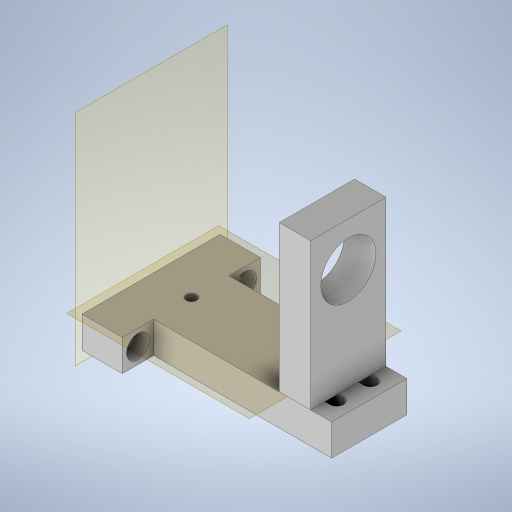
# Autodesk Inventor part: AdapterBracket
Saved by Autodesk Inventor 2024 (Build 280153000, 153)
## iProperties
Created: 2026-02-24
Part Number: AdapterBracket
Material: Generic
Document SubType Name: Modeling
Designer: nvladi
Density: 1 g/cm^3
Appearance: Default
Author: nvladi
Autodesk Inventor part; units mm, degrees
ref_plane "YZ Plane" through (0, 0, 0) normal (1, 0, 0) x (0, 1, 0)
ref_plane "XZ Plane" through (0, 0, 0) normal (0, 1, 0) x (-1, 0, 0)
ref_plane "Work Plane1" through (0, 0, 0) normal (0, 0, 1) x (1, 0, 0)
sketch "Sketch1" plane through (0, 0, 0) normal (0, 0, 1) x (1, 0, 0)
  line L0 (2, 95.25) -> (68, 95.25)
  line L1 (2, 80.25) -> (68, 80.25)
  line L2 (2, 0) -> (2, 95.25)
  line L3 (68, 95.25) -> (68, 0)
  point P0 (0, 0)
  constraints: 8 end point, 2 horizontal, 2 vertical, 6 other
ref_plane "Work Plane2" through (12.0686, 8.3392, 79.2624) normal (0, 0, 1) x (1, 0, 0)
extrude "Extrusion1" add sketch "Sketch1" along normal up to surface (79.2624 mm away)
sketch "Sketch2" plane through (2, 95.25, 79.2624) normal (0, 0, 1) x (1, 0, 0)
  line L0 (66, -15) -> (66, 0) projected
  line L1 (66, 0) -> (0, 0) projected
  line L2 (66, -15) -> (51, -15)
  line L3 (51, -15) -> (51, 0)
  line L4 (51, 0) -> (66, 0)
  line L5 (66, 0) -> (66, -15)
  line L6 (0, 0) -> (0, -15) projected
  line L7 (0, -15) -> (15, -15)
  line L8 (15, -15) -> (15, 0)
  line L9 (15, 0) -> (0, 0)
  line L10 (0, 0) -> (0, -15)
  point P0 (-2, -95.25)
  dimension "d2" = 15
  dimension "d3" = 15
  constraints: 16 end point, 4 parallel, 2 horizontal, 2 perpendicular, 2 point on line
  measures "d2" distance of L3.end L4.end
  measures "d3" distance of L9.end L8.end
extrude "Extrusion2" cut sketch "Sketch2" against normal blind 60
sketch "Sketch4" plane through (2, 95.25, 19.2624) normal (0, 0, 1) x (1, 0, 0)
  line L0 (66, -15) -> (51, -15) projected
  line L1 (66, 0) -> (66, -15) projected
  line L2 (51, 0) -> (66, 0) projected
  line L3 (51, -15) -> (51, 0) projected
  line L4 (15, -15) -> (0, -15) projected
  line L5 (0, -15) -> (0, 0) projected
  line L6 (15, 0) -> (15, -15) projected
  line L7 (0, 0) -> (15, 0) projected
  point P0 (-2, -95.25)
  point P1 (58.5, -7.5)
  point P2 (7.5, -7.5)
hole "Hole1" at (60.5, 87.75, 19.2624) at (9.5, 87.75, 19.2624) direction (0, 0, -1) diameter 6.6 end through all counterbore diameter 11 counterbore depth 6.8 clearance for "Socket Head Cap Screw ISO 4762" size "M6" standard "ISO"
sketch "Sketch5" plane through (2, 95.25, 0) normal (0, 1, 0) x (1, 0, 0)
  line L0 (51, -79.2624) -> (51, -19.2624) projected
  line L1 (15, -19.2624) -> (15, -79.2624) projected
  line L2 (15, -79.2624) -> (51, -79.2624) projected
  line L3 (51, -79.2624) -> (15, -79.2624)
  line L4 (15, -79.2624) -> (15, -94.2624)
  line L5 (15, -94.2624) -> (51, -94.2624)
  line L6 (51, -94.2624) -> (51, -79.2624)
  point P0 (-2, 0)
  dimension "d13" = 15
  constraints: 8 end point, 2 parallel, 1 horizontal, 1 perpendicular
  measures "d13" distance of L4.end L3.end
extrude "Extrusion3" add sketch "Sketch5" against normal blind 85
sketch "Sketch6" plane through (17, 95.25, 94.2624) normal (0, 0, 1) x (1, 0, 0)
  circle A0 centre (18, -64) radius 25
  circle A1 centre (18, -64) radius 13.1445
  point P0 (-17, -95.25)
  dimension "d16" = 26.289
  constraints: 2 centre point, 1 coincident, 2 other
  measures "d16" diameter of A1
extrude "Extrusion4" cut sketch "Sketch6" against normal up to surface (15 mm away) contours A1
sketch "Sketch7" plane through (2, 95.25, 0) normal (0, 1, 0) x (1, 0, 0)
  line L0 (66, 0) -> (0, 0) projected
  line L1 (51, -94.2624) -> (51, -19.2624) projected
  line L2 (15, -19.2624) -> (15, -94.2624) projected
  line L3 (15, -94.2624) -> (51, -94.2624) projected
  line L4 (51, -94.2624) -> (51, -19.2624) projected
  line L5 (51, -19.2624) -> (66, -19.2624) projected
  line L6 (66, 0) -> (66, -19.2624) projected
  line L7 (66, 0) -> (0, 0) projected
  line L8 (0, 0) -> (0, -19.2624) projected
  line L9 (0, -19.2624) -> (15, -19.2624) projected
  point P0 (-2, 0)
  point P1 (33, -19.2624)
  point P2 (33, -69.2624)
  dimension "d19" = 50
  constraints: 1 other
  measures "d19" distance of point (33, -69.262) point (33, -19.262)
hole "Hole2" at (35, 95.25, 19.2624) at (35, 95.25, 69.2624) direction (0, -1, 0) diameter 4.9784 depth 19.05 tip angle 118 thread size "1/4-20 UNC" class "2B" standard "ANSI Unified Screw Threads"
ref_plane "Work Plane3" through (2, 80.25, 0) normal (0, -1, 0) x (1, 0, 0)
split body "Split1" result two bodies by plane through (2, 80.25, 0) normal (0, -1, 0) first body at (35.5281, 68.2662, 93.7624)
sketch "Sketch8" plane through (17, 95.25, 94.2624) normal (0, 0, 1) x (1, 0, 0)
  line L0 (0, -15) -> (36, -15) projected
  line L1 (36, 0) -> (36, -15) projected
  line L2 (0, 0) -> (36, 0) projected
  line L3 (0, 0) -> (0, -15) projected
  point P0 (-17, -95.25)
extrude "Extrusion5" add sketch "Sketch8" along normal blind 10 bodies 3
sketch "Sketch10" plane through (17, 80.25, 94.2624) normal (0, 1, 0) x (1, 0, 0)
  line L0 (0, 0) -> (36, 0) projected
  line L1 (36, 0) -> (36, 15) projected
  line L2 (36, 15) -> (0, 15) projected
  line L3 (0, 15) -> (0, 0) projected
  point P0 (-17, 94.2624)
  point P1 (10, 7.5)
  point P2 (26, 7.5)
  point P3 (36, 7.5)
  dimension "d30" = 10
  dimension "d31" = 10
  constraints: 1 midpoint
  measures "d30" distance from line of point (10, 7.5) L3
  measures "d31" distance of point (26, 7.5) point (36, 7.5)
hole "Hole3" at (27, 80.25, 86.7624) at (43, 80.25, 86.7624) direction (0, -1, 0) diameter 4.917 depth 17.1 tip angle 118 bodies 2 thread size "M6x1" class "6H" standard "ISO Metric profile"
sketch "Sketch11" plane through (2, 95.25, 0) normal (0, 1, 0) x (1, 0, 0)
  circle A0 centre (41, -86.7624) radius 2.4585 projected
  circle A1 centre (25, -86.7624) radius 2.4585 projected
  line L0 (41, -96.7624) -> (41, -76.7624) construction
  line L1 (46.5, -96.7624) -> (46.5, -76.7624)
  line L2 (35.5, -76.7624) -> (35.5, -96.7624)
  arc A2 (35.5, -96.7624) -> (46.5, -96.7624) centre (41, -96.7624) ccw
  arc A3 (46.5, -76.7624) -> (35.5, -76.7624) centre (41, -76.7624) ccw
  line L3 (25, -96.7624) -> (25, -76.7624) construction
  line L4 (30.5, -96.7624) -> (30.5, -76.7624)
  line L5 (19.5, -76.7624) -> (19.5, -96.7624)
  arc A4 (19.5, -96.7624) -> (30.5, -96.7624) centre (25, -96.7624) ccw
  arc A5 (30.5, -76.7624) -> (19.5, -76.7624) centre (25, -76.7624) ccw
  line L6 (41, -96.7624) -> (41, -76.7624) construction
  line L7 (44.2, -96.7624) -> (44.2, -76.7624)
  line L8 (37.8, -76.7624) -> (37.8, -96.7624)
  arc A6 (37.8, -96.7624) -> (44.2, -96.7624) centre (41, -96.7624) ccw
  arc A7 (44.2, -76.7624) -> (37.8, -76.7624) centre (41, -76.7624) ccw
  line L9 (25, -96.7624) -> (25, -76.7624) construction
  line L10 (28.2, -96.7624) -> (28.2, -76.7624)
  line L11 (21.8, -76.7624) -> (21.8, -96.7624)
  arc A8 (21.8, -96.7624) -> (28.2, -96.7624) centre (25, -96.7624) ccw
  arc A9 (28.2, -76.7624) -> (21.8, -76.7624) centre (25, -76.7624) ccw
  point P0 (-2, 0)
  dimension "d39" = 10
  dimension "d40" = 11
  dimension "d41" = 10
  dimension "d42" = 11
  dimension "d43" = 6.4
  dimension "d44" = 6.4
  constraints: 32 end point, 16 point on circle, 16 tangent, 8 centre point, 7 equal length, 4 midpoint, 1 vertical
  measures "d39" distance of A0.centre L0.end
  measures "d40" diameter of A3
  measures "d41" distance of A1.centre L3.end
  measures "d42" diameter of A5
  measures "d43" diameter of A7
  measures "d44" diameter of A9
extrude "Extrusion6" cut sketch "Sketch11" against normal up to surface (15 mm away) contours A0 | A1 | A6 L8 A7 L7 | A8 L11 A9 L10 bodies 3
extrude "Extrusion7" cut sketch "Sketch11" against normal blind 7 contours A0 | A1 | A2 L2 A3 L1 | A4 L5 A5 L4 | A6 L8 A7 L7 | A8 L11 A9 L10 bodies 3
body "Solid2"
body "Solid3"
